Autodesk Inventor part; units mm, degrees
(part 3 of 3)
sketch "Эскиз12" plane through (0, 36.5, 0) normal (0, 1, 0) x (1, 0, 0)
  arc A0 (46.0909, 86.4848) -> (42.0132, 88.5375) centre (0, 0) ccw
  line L0 (42.7346, 92.2321) -> (44.244, 93.7415) construction
  arc A1 (44.244, 93.7415) -> (43.9555, 95.3568) centre (43.5369, 94.4486) ccw construction
  arc A2 (43.9555, 95.3568) -> (21.2019, 102.8371) centre (0, 0) ccw construction
  arc A3 (21.2019, 102.8371) -> (20, 101.8577) centre (21, 101.8577) ccw construction
  line L1 (20, 101.8577) -> (20, 99) construction
  arc A4 (41.6155, 92.028) -> (20, 99) centre (0, 0) ccw construction
  arc A5 (41.6155, 92.028) -> (42.7346, 92.2321) centre (42.0275, 92.9392) ccw construction
  line L2 (23.5, 96.5872) -> (23.5, 92.2976) construction
  arc A6 (25, 94.2341) -> (23.5, 92.2976) centre (25.5, 92.2976) ccw construction
  arc A7 (25, 94.2341) -> (27.022, 95.4865) centre (24, 98.1071) ccw construction
  arc A8 (30.1851, 96.3839) -> (27.022, 95.4865) centre (29.2885, 93.521) ccw construction
  arc A9 (30.1851, 96.3839) -> (25.5511, 97.7146) centre (0, 0) ccw construction
  arc A10 (25, 94.2341) -> (25.8102, 94.5401) centre (24, 98.1071) ccw construction
  line L3 (20.5, 98.8977) -> (20.5, 47.4035) construction
  line L4 (21.4454, 47.6084) -> (23.5, 49.663) construction
  line L5 (23.5, 49.663) -> (23.5, 98.2281) construction
  arc A11 (-23.5, 96.5872) -> (-25.5511, 97.7146) centre (-24, 98.1071) ccw construction
  line L6 (-23.5, 98.2281) -> (-23.5, 49.663) construction
  line L7 (-23.5, 49.663) -> (-21.4454, 47.6084) construction
  line L8 (-20.5, 47.4035) -> (-20.5, 98.8977) construction
  arc A12 (-25.5511, 97.7146) -> (-30.1851, 96.3839) centre (0, 0) ccw construction
  arc A13 (-27.022, 95.4865) -> (-30.1851, 96.3839) centre (-29.2885, 93.521) ccw construction
  arc A14 (-27.022, 95.4865) -> (-25, 94.2341) centre (-24, 98.1071) ccw construction
  arc A15 (-23.5, 92.2976) -> (-25, 94.2341) centre (-25.5, 92.2976) ccw construction
  line L9 (-23.5, 96.5872) -> (-23.5, 92.2976) construction
  arc A16 (-42.7346, 92.2321) -> (-41.6155, 92.028) centre (-42.0275, 92.9392) ccw construction
  arc A17 (-20, 99) -> (-41.6155, 92.028) centre (0, 0) ccw construction
  line L10 (-20, 99) -> (-20, 101.8577) construction
  arc A18 (-20, 101.8577) -> (-21.2019, 102.8371) centre (-21, 101.8577) ccw construction
  arc A19 (-21.2019, 102.8371) -> (-43.9555, 95.3568) centre (0, 0) ccw construction
  arc A20 (-43.9555, 95.3568) -> (-44.244, 93.7415) centre (-43.5369, 94.4486) ccw construction
  line L11 (-44.244, 93.7415) -> (-42.7346, 92.2321) construction
  line L12 (-76.014, 34.2947) -> (-34.2947, 76.014) construction
  arc A21 (-34.2947, 76.014) -> (-34.2947, 83.085) centre (-37.8302, 79.5495) ccw construction
  line L13 (-34.2947, 83.085) -> (-38.3892, 87.1795) construction
  arc A22 (-37.7453, 90.4395) -> (-38.3892, 87.1795) centre (-36.975, 88.5938) ccw construction
  arc A23 (-27.022, 95.4865) -> (-25.8102, 94.5401) centre (-24, 98.1071) ccw construction
  arc A24 (-27.022, 95.4865) -> (-30.1851, 96.3839) centre (-29.2885, 93.521) ccw construction
  arc A25 (-30.1851, 96.3839) -> (-41.6155, 92.028) centre (0, 0) ccw construction
  arc A26 (-42.7346, 92.2321) -> (-41.6155, 92.028) centre (-42.0275, 92.9392) ccw construction
  line L14 (-42.7346, 92.2321) -> (-44.244, 93.7415) construction
  arc A27 (-43.9555, 95.3568) -> (-44.244, 93.7415) centre (-43.5369, 94.4486) ccw construction
  arc A28 (-43.9555, 95.3568) -> (-48.6481, 93.0503) centre (0, 0) ccw projected
  arc A29 (-48.6481, 93.0503) -> (-49.3795, 88.2704) centre (-47.2582, 90.3917) ccw projected
  line L15 (-49.3795, 88.2704) -> (-46.3155, 85.2064) construction
  arc A30 (-46.3155, 73.8927) -> (-46.3155, 85.2064) centre (-51.9723, 79.5495) ccw construction
  line L16 (-46.3155, 73.8927) -> (-73.8927, 46.3155) construction
  arc A31 (-85.2064, 46.3155) -> (-73.8927, 46.3155) centre (-79.5495, 51.9723) ccw construction
  line L17 (-85.2064, 46.3155) -> (-88.2704, 49.3795) construction
  arc A32 (-88.2704, 49.3795) -> (-93.0503, 48.6481) centre (-90.3917, 47.2582) ccw construction
  arc A33 (-93.0503, 48.6481) -> (-93.0503, -48.6481) centre (0, 0) ccw construction
  arc A34 (-93.0503, -48.6481) -> (-88.2704, -49.3795) centre (-90.3917, -47.2582) ccw construction
  line L18 (-88.2704, -49.3795) -> (-85.2064, -46.3155) construction
  arc A35 (-73.8927, -46.3155) -> (-85.2064, -46.3155) centre (-79.5495, -51.9723) ccw construction
  line L19 (-73.8927, -46.3155) -> (-46.3155, -73.8927) construction
  arc A36 (-46.3155, -85.2064) -> (-46.3155, -73.8927) centre (-51.9723, -79.5495) ccw construction
  line L20 (-46.3155, -85.2064) -> (-49.3795, -88.2704) construction
  arc A37 (-49.3795, -88.2704) -> (-48.6481, -93.0503) centre (-47.2582, -90.3917) ccw construction
  arc A38 (-48.6481, -93.0503) -> (-45.42, -94.668) centre (0, 0) ccw construction
  arc A39 (-45.42, -94.668) -> (-43.0355, -94.1655) centre (-44.5548, -92.8648) ccw construction
  line L21 (-43.0355, -94.1655) -> (-18.3802, -65.3664) construction
  arc A40 (-17.477, -64.7643) -> (-18.3802, -65.3664) centre (-16.8609, -66.6671) ccw construction
  line L22 (-17.477, -64.7643) -> (-0.6161, -59.3045) construction
  arc A41 (0.6161, -59.3045) -> (-0.6161, -59.3045) centre (0, -61.2072) ccw construction
  line L23 (0.6161, -59.3045) -> (17.477, -64.7643) construction
  arc A42 (18.3802, -65.3664) -> (17.477, -64.7643) centre (16.8609, -66.6671) ccw construction
  line L24 (18.3802, -65.3664) -> (43.0355, -94.1655) construction
  arc A43 (43.0355, -94.1655) -> (45.42, -94.668) centre (44.5548, -92.8648) ccw construction
  arc A44 (45.42, -94.668) -> (48.6481, -93.0503) centre (0, 0) ccw construction
  arc A45 (48.6481, -93.0503) -> (49.3795, -88.2704) centre (47.2582, -90.3917) ccw construction
  line L25 (49.3795, -88.2704) -> (46.3155, -85.2064) construction
  arc A46 (46.3155, -73.8927) -> (46.3155, -85.2064) centre (51.9723, -79.5495) ccw construction
  line L26 (46.3155, -73.8927) -> (73.8927, -46.3155) construction
  arc A47 (85.2064, -46.3155) -> (73.8927, -46.3155) centre (79.5495, -51.9723) ccw construction
  line L27 (85.2064, -46.3155) -> (88.2704, -49.3795) construction
  arc A48 (88.2704, -49.3795) -> (93.0503, -48.6481) centre (90.3917, -47.2582) ccw construction
  arc A49 (93.0503, -48.6481) -> (93.0503, 48.6481) centre (0, 0) ccw construction
  arc A50 (93.0503, 48.6481) -> (88.2704, 49.3795) centre (90.3917, 47.2582) ccw construction
  line L28 (88.2704, 49.3795) -> (85.2064, 46.3155) construction
  arc A51 (73.8927, 46.3155) -> (85.2064, 46.3155) centre (79.5495, 51.9723) ccw construction
  line L29 (73.8927, 46.3155) -> (46.3155, 73.8927) construction
  arc A52 (46.3155, 85.2064) -> (46.3155, 73.8927) centre (51.9723, 79.5495) ccw construction
  line L30 (46.3155, 85.2064) -> (49.3795, 88.2704) construction
  arc A53 (49.3795, 88.2704) -> (48.6481, 93.0503) centre (47.2582, 90.3917) ccw projected
  arc A54 (48.6481, 93.0503) -> (43.9555, 95.3568) centre (0, 0) ccw construction
  arc A55 (44.244, 93.7415) -> (43.9555, 95.3568) centre (43.5369, 94.4486) ccw construction
  line L31 (44.244, 93.7415) -> (42.7346, 92.2321) construction
  arc A56 (41.6155, 92.028) -> (42.7346, 92.2321) centre (42.0275, 92.9392) ccw construction
  arc A57 (41.6155, 92.028) -> (30.1851, 96.3839) centre (0, 0) ccw construction
  arc A58 (30.1851, 96.3839) -> (27.022, 95.4865) centre (29.2885, 93.521) ccw construction
  arc A59 (25.8102, 94.5401) -> (27.022, 95.4865) centre (24, 98.1071) ccw construction
  arc A60 (38.3892, 87.1795) -> (37.7453, 90.4395) centre (36.975, 88.5938) ccw construction
  line L32 (38.3892, 87.1795) -> (34.2947, 83.085) construction
  arc A61 (34.2947, 83.085) -> (34.2947, 76.014) centre (37.8302, 79.5495) ccw construction
  line L33 (34.2947, 76.014) -> (76.014, 34.2947) construction
  line L34 (76.014, -34.2947) -> (37.1244, -73.1843) construction
  arc A62 (34.1909, -73.0707) -> (37.1244, -73.1843) centre (35.7102, -71.7701) ccw construction
  line L35 (34.1909, -73.0707) -> (25.4187, -62.8242) construction
  arc A63 (24.842, -61.8893) -> (25.4187, -62.8242) centre (28.1154, -60.5155) ccw construction
  line L36 (24.842, -61.8893) -> (23.8313, -59.4808) construction
  arc A64 (23.8313, -59.4808) -> (21.0049, -57.3328) centre (20.5578, -60.8546) ccw construction
  line L37 (21.0049, -57.3328) -> (15.1585, -56.5907) construction
  arc A65 (14.5119, -56.4463) -> (15.1585, -56.5907) centre (15.6055, -53.069) ccw construction
  line L38 (14.5119, -56.4463) -> (0.6161, -51.9466) construction
  arc A66 (0.6161, -51.9466) -> (-0.6161, -51.9466) centre (0, -53.8493) ccw construction
  line L39 (-0.6161, -51.9466) -> (-14.5119, -56.4463) construction
  arc A67 (-15.1585, -56.5907) -> (-14.5119, -56.4463) centre (-15.6055, -53.069) ccw construction
  line L40 (-15.1585, -56.5907) -> (-21.0049, -57.3328) construction
  arc A68 (-21.0049, -57.3328) -> (-23.8313, -59.4808) centre (-20.5578, -60.8546) ccw construction
  line L41 (-23.8313, -59.4808) -> (-24.842, -61.8893) construction
  arc A69 (-25.4187, -62.8242) -> (-24.842, -61.8893) centre (-28.1154, -60.5155) ccw construction
  line L42 (-25.4187, -62.8242) -> (-34.1909, -73.0707) construction
  arc A70 (-37.1244, -73.1843) -> (-34.1909, -73.0707) centre (-35.7102, -71.7701) ccw construction
  line L43 (-37.1244, -73.1843) -> (-76.014, -34.2947) construction
  arc A71 (76.014, 34.2947) -> (83.085, 34.2947) centre (79.5495, 37.8302) ccw construction
  line L44 (83.085, 34.2947) -> (87.1795, 38.3892) construction
  arc A72 (90.4395, 37.7453) -> (87.1795, 38.3892) centre (88.5938, 36.975) ccw construction
  arc A73 (90.4395, -37.7453) -> (90.4395, 37.7453) centre (0, 0) ccw construction
  arc A74 (87.1795, -38.3892) -> (90.4395, -37.7453) centre (88.5938, -36.975) ccw construction
  line L45 (87.1795, -38.3892) -> (83.085, -34.2947) construction
  arc A75 (83.085, -34.2947) -> (76.014, -34.2947) centre (79.5495, -37.8302) ccw construction
  circle A76 centre (79.5495, -37.8302) radius 1.6 construction
  circle A77 centre (37.8302, 79.5495) radius 1.6 construction
  circle A78 centre (79.5495, 37.8302) radius 1.6 construction
  circle A79 centre (20.5578, -60.8546) radius 1.55 construction
  circle A80 centre (37.8302, -79.5495) radius 1.6 construction
  arc A81 (-76.014, -34.2947) -> (-83.085, -34.2947) centre (-79.5495, -37.8302) ccw construction
  line L46 (-83.085, -34.2947) -> (-87.1795, -38.3892) construction
  arc A82 (-90.4395, -37.7453) -> (-87.1795, -38.3892) centre (-88.5938, -36.975) ccw construction
  arc A83 (-90.4395, 37.7453) -> (-90.4395, -37.7453) centre (0, 0) ccw construction
  arc A84 (-87.1795, 38.3892) -> (-90.4395, 37.7453) centre (-88.5938, 36.975) ccw construction
  line L47 (-87.1795, 38.3892) -> (-83.085, 34.2947) construction
  arc A85 (-83.085, 34.2947) -> (-76.014, 34.2947) centre (-79.5495, 37.8302) ccw construction
  circle A86 centre (-37.8302, 79.5495) radius 1.6 construction
  circle A87 centre (-79.5495, 37.8302) radius 1.6 construction
  circle A88 centre (-79.5495, -37.8302) radius 1.6 construction
  circle A89 centre (-20.5578, -60.8546) radius 1.55 construction
  circle A90 centre (-37.8302, -79.5495) radius 1.6 construction
  arc A91 (41.4241, 88.8147) -> (41.4975, 92.0812) centre (45.1111, 90.3659) ccw construction
  arc A92 (41.6155, 92.028) -> (20, 99) centre (0, 0) ccw projected
  arc A93 (41.6155, 92.028) -> (41.4975, 92.0812) centre (0, 0) ccw construction
  arc A94 (41.1291, 90.7454) -> (41.1834, 89.6088) centre (45.1111, 90.3659) ccw
  arc A95 (39.9288, 92.7723) -> (20, 99) centre (0, 0) ccw construction
  arc A96 (41.1291, 90.7454) -> (39.9288, 92.7723) centre (39.1381, 90.9352) ccw
  arc A97 (85.9577, 47.0668) -> (47.0668, 85.9577) centre (0, 0) ccw construction
  arc A98 (41.4241, 88.8147) -> (85.9577, 47.0668) centre (0, 0) ccw construction
  arc A99 (41.1834, 89.6088) -> (42.0132, 88.5375) centre (42.6562, 89.8927) ccw
  line L48 (46.3155, 85.2064) -> (49.3795, 88.2704) construction
  line L49 (49.3795, 88.2704) -> (47.8571, 86.7479)
  arc A100 (46.0909, 86.4848) -> (47.8571, 86.7479) centre (46.7964, 87.8086) ccw
  arc A101 (48.6481, 93.0503) -> (43.9555, 95.3568) centre (0, 0) ccw projected
  arc A102 (48.6481, 93.0503) -> (43.9555, 95.3568) centre (0, 0) ccw
  line L50 (43.9555, 95.3568) -> (39.9288, 92.7723)
  line L51 (2.9667, 51) -> (2.9667, 97.4549) construction
  arc A103 (2.9667, 97.4549) -> (-2.9667, 97.4549) centre (0, 0) ccw construction
  line L52 (-2.9667, 97.4549) -> (-2.9667, 51) construction
  line L53 (0, 46) -> (0, 97.5) construction
  arc A104 (20.4598, 95.3292) -> (-20.4598, 95.3292) centre (0, 0) ccw construction
  arc A105 (49.3795, 88.2704) -> (48.6481, 93.0503) centre (47.2582, 90.3917) ccw
  line L54 (-43.9555, 95.3568) -> (-39.9288, 92.7723)
  arc A106 (-41.1834, 89.6088) -> (-41.1291, 90.7454) centre (-45.1111, 90.3659) ccw
  arc A107 (-39.9288, 92.7723) -> (-41.1291, 90.7454) centre (-39.1381, 90.9352) ccw
  arc A108 (-42.0132, 88.5375) -> (-41.1834, 89.6088) centre (-42.6562, 89.8927) ccw
  arc A109 (-42.0132, 88.5375) -> (-46.0909, 86.4848) centre (0, 0) ccw
  line L55 (-49.3795, 88.2704) -> (-47.8571, 86.7479)
  arc A110 (-47.8571, 86.7479) -> (-46.0909, 86.4848) centre (-46.7964, 87.8086) ccw
  arc A111 (-43.9555, 95.3568) -> (-48.6481, 93.0503) centre (0, 0) ccw construction
  arc A112 (-43.9555, 95.3568) -> (-48.6481, 93.0503) centre (0, 0) ccw construction
  arc A113 (-25.8102, 94.5401) -> (-37.7453, 90.4395) centre (0, 0) ccw projected
  arc A114 (37.7453, 90.4395) -> (25.8102, 94.5401) centre (0, 0) ccw projected
  line L56 (-2.9667, 51) -> (2.9667, 51) projected
  circle A115 centre (45.1111, 90.3659) radius 1.9
  circle A116 centre (-45.1111, 90.3659) radius 1.9
  arc A117 (-25.5511, 97.7146) -> (-23.5, 96.5872) centre (-24, 98.1071) ccw projected
  arc A118 (23.5, 96.5872) -> (25.5511, 97.7146) centre (24, 98.1071) ccw projected
  point P0 (20.7476, 95.7786)
  dimension "d170" = 196
  dimension "d171" = 8
  dimension "d172" = 2
  dimension "d173" = 1.5
  dimension "d174" = 1.5
  dimension "d175" = 105
  dimension "d178" = 3.8
  constraints: 44 point on circle, 20 centre point, 12 symmetric about line, 10 end point, 8 tangent, 3 point on line, 2 coincident, 1 collinear, 10 other
  measures "d170" diameter of A0
  measures "d171" diameter of A91
  measures "d172" radius of A96
  measures "d173" radius of A99
  measures "d174" radius of A100
  measures "d175" radius of A102
  measures "d178" diameter of A115
extrude "Выдавливание18" add sketch "Эскиз12" along normal blind 0.3 and the other way blind 34.5
fillet "Сопряжение4" radius 2 1 edges at (0.1642, 2, -51)
